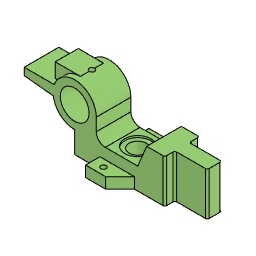
Exercise-13 v1 (Autodesk Fusion 360 design; units mm, degrees)
Autodesk Fusion 360 part; units mm, degrees
sketch "Sketch1" plane through (0, 0, 0) normal (0, 0, 1) x (1, 0, 0)
  line L0 (50, -24) -> (-50, -24)
  line L1 (-50, -24) -> (-50, 24)
  line L2 (-50, 24) -> (50, 24)
  line L3 (50, 24) -> (50, -24)
  line L4 (50, -24) -> (-50, 24) construction
  line L5 (-50, -24) -> (50, 24) construction
  dimension "d1" = 100
  dimension "d2" = 48
  constraint horizontal L0
  constraint perpendicular L0 L1
  constraint parallel L0 L2
  constraint parallel L1 L3
  constraint coincident L4 origin
  constraint coincident L5 origin
  measures "d1" distance of L1.end L2.end
  measures "d2" distance of L0.end L1.end
extrude "Extrude1" add sketch "Sketch1" along normal blind 30
sketch "Sketch2" plane through (0, 0, 0) normal (0, 1, 0) x (1, 0, 0)
  line L0 (50, 0) -> (50, -30)
  line L1 (50, 0) -> (-50, 0)
  line L2 (-50, -30) -> (50, -30)
  line L3 (-50, 0) -> (-50, -30)
  line L4 (50, 0) -> (75, 0)
  line L5 (75, 0) -> (75, -60)
  line L6 (75, -60) -> (50, -60)
  line L7 (50, -60) -> (50, 0)
  line L8 (75, -60) -> (120, -60)
  line L9 (120, -60) -> (120, 0)
  line L10 (120, 0) -> (75, 0)
  line L11 (75, 0) -> (75, -60)
  line L12 (50, -60) -> (37.5, -30)
  circle A0 centre (-50, -60) radius 30
  circle A1 centre (-50, -60) radius 20
  line L13 (-15, 0) -> (33, 0)
  line L14 (33, 0) -> (33, -15)
  line L15 (33, -15) -> (-15, -15)
  line L16 (-15, -15) -> (-15, 0)
  line L17 (-50, -60) -> (-50, -70)
  line L18 (-50, -70) -> (-120, -70)
  line L19 (-120, -70) -> (-120, -60)
  line L20 (-50, -60) -> (-50, -52.5)
  line L21 (-50, -52.5) -> (-120, -60)
  line L22 (-50, -90) -> (-85, -90)
  line L23 (-85, -90) -> (-85, -70)
  line L24 (-20, -60) -> (-20, -30)
  dimension "d5" = 25
  dimension "d6" = 60
  dimension "d7" = 45
  dimension "d8" = 60
  dimension "d9" = 60
  dimension "d10" = 40
  dimension "d11" = 48
  dimension "d12" = 15
  dimension "d13" = 10
  dimension "d14" = 70
  dimension "d15" = 10
  dimension "d16" = 7.5
  dimension "d17" = 35
  dimension "d18" = 12.5
  constraint horizontal L4
  constraint vertical L5
  constraint horizontal L6
  constraint vertical L7
  constraint coincident L0.start L1.start
  constraint horizontal L8
  constraint vertical L9
  constraint horizontal L10
  constraint vertical L11
  constraint coincident L2 L12.end
  constraint coincident L2.start A0
  constraint concentric A0 A1
  constraint horizontal L13
  constraint vertical L14
  constraint horizontal L15
  constraint vertical L16
  constraint coincident L1 L13.start
  constraint coincident A0.centre A1.centre
  constraint vertical L17
  constraint perpendicular L17 L18
  constraint perpendicular L18 L19
  constraint parallel L17 L20
  constraint coincident A0 L22.start
  constraint tangent A0 L22
  constraint parallel L18 L22
  constraint midpoint L18 L23.end
  constraint perpendicular L18 L23
  constraint coincident A0 L24.start
  constraint coincident L2 L24.end
  constraint tangent A0 L24
  constraint perpendicular L2 L24
  measures "d5" distance of L0.start L4.end
  measures "d6" distance of L0.start L6.end
  measures "d7" distance of L5.end L8.end
  measures "d8" distance of L5.end L4.end
  measures "d9" diameter of A0
  measures "d10" diameter of A1
  measures "d11" distance of L13.start L13.end
  measures "d12" distance of L13.start L15.end
  measures "d13" distance of A0.centre L17.end
  measures "d14" distance of L17.end L18.end
  measures "d15" distance of L18.end L19.end
  measures "d16" distance of A0.centre L20.end
  measures "d17" distance of L1.end L13.start
  measures "d18" distance of L0.end L12.end
extrude "Extrude2" add sketch "Sketch2" along normal mid plane 48 contours L0 L4 L5 L6 L7 L11 | L2 L7 L12 | L2 A0 L24 | A0 A1 L18 L21 | A0 A1 L18 L21 | A0 L18 L19 L21
extrude "Extrude3" add sketch "Sketch2" along normal mid plane 20 contours L5 L8 L9 L10 L11
extrude "Extrude4" add sketch "Sketch2" along normal mid plane 32 contours A0 L18 L22 L23
extrude "Extrude5" add sketch "Sketch2" against normal blind 20 from surface at -24 contours L1 L13 L14 L15 L16
sketch "Sketch3" plane through (0, 0, 15) normal (0, 0, 1) x (-1, 0, 0)
  line L0 (-33, 24) -> (15, 24)
  line L1 (15, 24) -> (15, 44)
  line L2 (15, 44) -> (-33, 44)
  line L3 (-33, 44) -> (-33, 24)
  line L4 (-33, 24) -> (-3.3997, 53.6003)
  line L5 (-33, 24) -> (8.8612, 24) construction
  circle A0 centre (0, 34) radius 3.75
  dimension "d28" = 45
  dimension "d29" = 7.5
  dimension "d30" = 15
  constraint horizontal L5
  constraint coincident L0.start L3.end
  measures "d28" angle of L4 L5
  measures "d29" diameter of A0
  measures "d30" distance of L1 A0.centre
extrude "Extrude6" cut sketch "Sketch3" against normal blind 40 contours L2 L3 L4 | A0
extrude "Extrude7" add sketch "Sketch2" along normal blind 20 from surface at 24 contours L1 L13 L14 L15 L16
mirror "Mirror1" about plane through (0, 0, 0) normal (0, 1, 0) of "Extrude6"
hole "Hole1" at (-50, 0, 90) direction (0, 0, -1) diameter 7.5 depth 15 tip angle 180
hole "Hole2" at (13.5, 0, 30) direction (0, 0, -1) diameter 24 end through all counterbore diameter 36 counterbore depth 2.5
fillet "Fillet1" radius 12.5 1 edges at (-20, 0, 30)
fillet "Fillet2" radius 2.5 6 edges at (75, -10, 30) (120, -10, 30) (120, 10, 30) (75, -24, 30) (75, 24, 30) (75, 10, 30)
